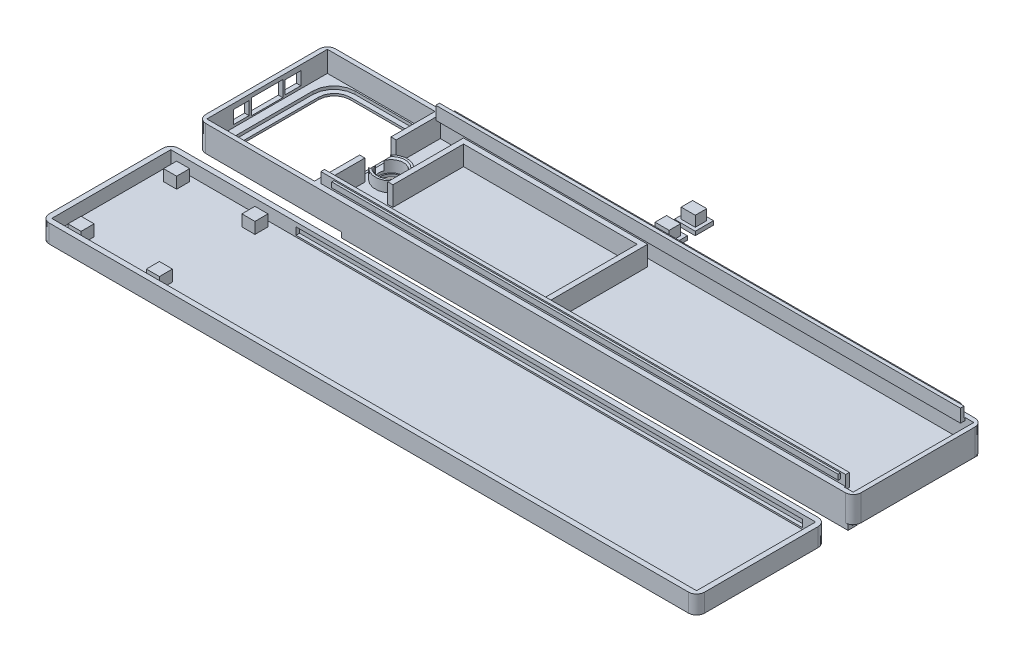
MeetingLight-Enclosure-v11 (Autodesk Fusion 360 design; units mm, degrees)
Autodesk Fusion 360 part; units mm, degrees
sketch "TRAY_Shell" plane through (0, 0, 0) normal (0, 0, 1) x (1, 0, 0)
  line L0 (0, 0) -> (251, 0)
  line L1 (251, 0) -> (251, 49.6)
  line L2 (251, 49.6) -> (0, 49.6)
  line L3 (0, 49.6) -> (0, 0)
  dimension "d26" = 251
  dimension "d27" = 49.6
  constraint coincident L0.start L3.end
  measures "d26" horizontal distance of L0.start L0.end
  measures "d27" vertical distance of L0.start L2.end
extrude "TRAY_Shell (1)" add sketch "TRAY_Shell" along normal blind 7 makes body 1
fillet "TRAY_CornerFillet" radius 3 4 edges at (0, 49.6, 3.5) (251, 49.6, 3.5) (251, 0, 3.5) (0, 0, 3.5) on bodies 1
sketch "TRAY_Cavity" plane through (0, 0, 0) normal (0, 0, 1) x (1, 0, 0)
  line L0 (2, 2) -> (249, 2)
  line L1 (249, 2) -> (249, 47.6)
  line L2 (249, 47.6) -> (2, 47.6)
  line L3 (2, 47.6) -> (2, 2)
  dimension "d32" = 247
  dimension "d33" = 45.6
  dimension "d34" = 2
  dimension "d35" = 2
  constraint horizontal L0
  constraint vertical L1
  measures "d32" horizontal distance of L0.start L0.end
  measures "d33" vertical distance of L0.start L2.end
  measures "d34" horizontal distance of origin L0.start
  measures "d35" vertical distance of origin L0.start
extrude "TRAY_Cavity (1)" cut sketch "TRAY_Cavity" along normal blind 5 from surface at 2 bodies 1
sketch "TRAY_ClampPads" plane through (0, 0, 0) normal (0, 0, 1) x (1, 0, 0)
  line L0 (6.24, 4) -> (11.24, 4)
  line L1 (11.24, 4) -> (11.24, 9)
  line L2 (11.24, 9) -> (6.24, 9)
  line L3 (6.24, 9) -> (6.24, 4)
  line L4 (36.24, 4) -> (41.24, 4)
  line L5 (41.24, 4) -> (41.24, 9)
  line L6 (41.24, 9) -> (36.24, 9)
  line L7 (36.24, 9) -> (36.24, 4)
  line L8 (6.24, 40.6) -> (11.24, 40.6)
  line L9 (11.24, 40.6) -> (11.24, 45.6)
  line L10 (11.24, 45.6) -> (6.24, 45.6)
  line L11 (6.24, 45.6) -> (6.24, 40.6)
  line L12 (36.24, 40.6) -> (41.24, 40.6)
  line L13 (41.24, 40.6) -> (41.24, 45.6)
  line L14 (41.24, 45.6) -> (36.24, 45.6)
  line L15 (36.24, 45.6) -> (36.24, 40.6)
extrude "TRAY_ClampPads (1)" add sketch "TRAY_ClampPads" along normal blind 4.33 from surface at 2 bodies 1
sketch "TRAY_SnapGroove" plane through (0, 0, 0) normal (0, 0, 1) x (1, 0, 0)
  line L0 (50, 0.65) -> (244, 0.65)
  line L1 (244, 0.65) -> (244, 2)
  line L2 (244, 2) -> (50, 2)
  line L3 (50, 2) -> (50, 0.65)
  line L4 (50, 47.6) -> (244, 47.6)
  line L5 (244, 47.6) -> (244, 48.95)
  line L6 (244, 48.95) -> (50, 48.95)
  line L7 (50, 48.95) -> (50, 47.6)
extrude "TRAY_SnapGroove (1)" cut sketch "TRAY_SnapGroove" along normal blind 2.8 from surface at 2.6 bodies 1
sketch "LID_Shell" plane through (0, 0, 0) normal (0, 0, 1) x (1, 0, 0)
  line L0 (0, 0) -> (251, 0)
  line L1 (251, 0) -> (251, 49.6)
  line L2 (251, 49.6) -> (0, 49.6)
  line L3 (0, 49.6) -> (0, 0)
  dimension "d47" = 251
  dimension "d48" = 49.6
  constraint coincident L0.start L3.end
  measures "d47" horizontal distance of L0.start L0.end
  measures "d48" vertical distance of L0.start L2.end
extrude "LID_Shell (1)" add sketch "LID_Shell" along normal blind 10 separate body makes body 2
fillet "LID_CornerFillet" radius 3 4 edges at (0, 49.6, 5) (251, 49.6, 5) (251, 0, 5) (0, 0, 5) on bodies 2
sketch "LID_Cavity" plane through (0, 0, 0) normal (0, 0, 1) x (1, 0, 0)
  line L0 (1.7, 1.7) -> (249.3, 1.7)
  line L1 (249.3, 1.7) -> (249.3, 47.9)
  line L2 (249.3, 47.9) -> (1.7, 47.9)
  line L3 (1.7, 47.9) -> (1.7, 1.7)
  dimension "d53" = 247.6
  dimension "d54" = 46.2
  dimension "d55" = 1.7
  dimension "d56" = 1.7
  measures "d53" horizontal distance of L0.start L0.end
  measures "d54" vertical distance of L0.start L2.end
  measures "d55" horizontal distance of origin L0.start
  measures "d56" vertical distance of origin L0.start
extrude "LID_Cavity (1)" cut sketch "LID_Cavity" along normal blind 8 from surface at 2 bodies 2
sketch "SCREEN_GlassRecess" plane through (0, 0, 0) normal (0, 0, 1) x (1, 0, 0)
  line L0 (6.75, 4.08) -> (40.25, 4.08)
  line L1 (40.25, 4.08) -> (40.25, 45.52)
  line L2 (40.25, 45.52) -> (6.75, 45.52)
  line L3 (6.75, 45.52) -> (6.75, 4.08)
extrude "SCREEN_GlassRecess (1)" cut sketch "SCREEN_GlassRecess" along normal blind 0.84 bodies 2
fillet "SCREEN_GlassRecess_R" radius 6 4 edges at (40.25, 45.52, 0.42) (6.75, 45.52, 0.42) (40.25, 4.08, 0.42) (6.75, 4.08, 0.42) on bodies 2
sketch "SCREEN_BodyOpening" plane through (0, 0, 0) normal (0, 0, 1) x (1, 0, 0)
  line L0 (4.75, 2.25) -> (42.25, 2.25)
  line L1 (42.25, 2.25) -> (42.25, 47.35)
  line L2 (42.25, 47.35) -> (4.75, 47.35)
  line L3 (4.75, 47.35) -> (4.75, 2.25)
extrude "SCREEN_BodyOpening (1)" cut sketch "SCREEN_BodyOpening" along normal blind 1.2 from surface at 0.84 bodies 2
fillet "SCREEN_BodyOpening_R" radius 8 4 edges at (42.25, 2.25, 1.42) (4.75, 2.25, 1.42) (4.75, 47.35, 1.42) (42.25, 47.35, 1.42) on bodies 2
sketch "SCREEN_XStop" plane through (0, 0, 0) normal (0, 0, 1) x (1, 0, 0)
  line L0 (42.94, 1.7) -> (44.94, 1.7)
  line L1 (44.94, 1.7) -> (44.94, 19)
  line L2 (44.94, 19) -> (42.94, 19)
  line L3 (42.94, 19) -> (42.94, 1.7)
  line L4 (42.94, 31) -> (44.94, 31)
  line L5 (44.94, 31) -> (44.94, 47.9)
  line L6 (44.94, 47.9) -> (42.94, 47.9)
  line L7 (42.94, 47.9) -> (42.94, 31)
extrude "SCREEN_XStop (1)" add sketch "SCREEN_XStop" along normal blind 8 from surface at 2 bodies 2
sketch "PAPER_LipFrontWall" plane through (0, 0, 0) normal (0, 0, 1) x (1, 0, 0)
  line L0 (54.99, 0) -> (249.01, 0)
  line L1 (249.01, 0) -> (249.01, 1.5)
  line L2 (249.01, 1.5) -> (54.99, 1.5)
  line L3 (54.99, 1.5) -> (54.99, 0)
extrude "PAPER_LipFrontWall (1)" add sketch "PAPER_LipFrontWall" against normal blind 2 bodies 2
sketch "PAPER_LipFrontShelf" plane through (0, 0, 0) normal (0, 0, 1) x (1, 0, 0)
  line L0 (54.99, 1.5) -> (249.01, 1.5)
  line L1 (249.01, 1.5) -> (249.01, 3.5)
  line L2 (249.01, 3.5) -> (54.99, 3.5)
  line L3 (54.99, 3.5) -> (54.99, 1.5)
extrude "PAPER_LipFrontShelf (1)" add sketch "PAPER_LipFrontShelf" along normal blind 0.8 from surface at -2 bodies 2
sketch "PAPER_LipBackWall" plane through (0, 0, 0) normal (0, 0, 1) x (1, 0, 0)
  line L0 (54.99, 48.1) -> (249.01, 48.1)
  line L1 (249.01, 48.1) -> (249.01, 49.6)
  line L2 (249.01, 49.6) -> (54.99, 49.6)
  line L3 (54.99, 49.6) -> (54.99, 48.1)
extrude "PAPER_LipBackWall (1)" add sketch "PAPER_LipBackWall" against normal blind 2 bodies 2
sketch "PAPER_LipBackShelf" plane through (0, 0, 0) normal (0, 0, 1) x (1, 0, 0)
  line L0 (54.99, 46.1) -> (249.01, 46.1)
  line L1 (249.01, 46.1) -> (249.01, 48.1)
  line L2 (249.01, 48.1) -> (54.99, 48.1)
  line L3 (54.99, 48.1) -> (54.99, 46.1)
extrude "PAPER_LipBackShelf (1)" add sketch "PAPER_LipBackShelf" along normal blind 0.8 from surface at -2 bodies 2
sketch "BAT_PocketWalls" plane through (0, 0, 0) normal (0, 0, 1) x (1, 0, 0)
  line L0 (56.7, 16) -> (58.7, 16)
  line L1 (58.7, 16) -> (58.7, 43.05)
  line L2 (58.7, 43.05) -> (56.7, 43.05)
  line L3 (56.7, 43.05) -> (56.7, 16)
  line L4 (56.7, 43.05) -> (127.2, 43.05)
  line L5 (127.2, 43.05) -> (127.2, 45.05)
  line L6 (127.2, 45.05) -> (56.7, 45.05)
  line L7 (56.7, 45.05) -> (56.7, 43.05)
  line L8 (125.2, 6.55) -> (127.2, 6.55)
  line L9 (127.2, 6.55) -> (127.2, 43.05)
  line L10 (127.2, 43.05) -> (125.2, 43.05)
  line L11 (125.2, 43.05) -> (125.2, 6.55)
  line L12 (56.7, 4.55) -> (127.2, 4.55)
  line L13 (127.2, 4.55) -> (127.2, 6.55)
  line L14 (127.2, 6.55) -> (56.7, 6.55)
  line L15 (56.7, 6.55) -> (56.7, 4.55)
extrude "BAT_PocketWalls (1)" add sketch "BAT_PocketWalls" along normal blind 7.5 from surface at 2 bodies 2
sketch "JOINT_RabbetFoot" plane through (0, 0, 0) normal (0, 0, 1) x (1, 0, 0)
  line L0 (45, 1) -> (246, 1)
  line L1 (246, 1) -> (246, 3.5)
  line L2 (246, 3.5) -> (45, 3.5)
  line L3 (45, 3.5) -> (45, 1)
  line L4 (45, 46.1) -> (246, 46.1)
  line L5 (246, 46.1) -> (246, 48.6)
  line L6 (246, 48.6) -> (45, 48.6)
  line L7 (45, 48.6) -> (45, 46.1)
extrude "JOINT_RabbetFoot (1)" add sketch "JOINT_RabbetFoot" along normal blind 1 from surface at 9 bodies 2
sketch "JOINT_RabbetLip" plane through (0, 0, 0) normal (0, 0, 1) x (1, 0, 0)
  line L0 (45, 2.1) -> (246, 2.1)
  line L1 (246, 2.1) -> (246, 3.5)
  line L2 (246, 3.5) -> (45, 3.5)
  line L3 (45, 3.5) -> (45, 2.1)
  line L4 (45, 46.1) -> (246, 46.1)
  line L5 (246, 46.1) -> (246, 47.5)
  line L6 (246, 47.5) -> (45, 47.5)
  line L7 (45, 47.5) -> (45, 46.1)
extrude "JOINT_RabbetLip (1)" add sketch "JOINT_RabbetLip" along normal blind 4 from surface at 10 bodies 2
sketch "IO_USB" plane through (0, 0, 0) normal (0, 0, 1) x (1, 0, 0)
  line L0 (-0.5, 18.8) -> (2, 18.8)
  line L1 (2, 18.8) -> (2, 30.8)
  line L2 (2, 30.8) -> (-0.5, 30.8)
  line L3 (-0.5, 30.8) -> (-0.5, 18.8)
  dimension "d97" = 12
  measures "d97" vertical distance of L0.start L2.end
extrude "IO_USB (1)" cut sketch "IO_USB" along normal blind 6 from surface at 2.5 bodies 2
sketch "IO_Btn1" plane through (0, 0, 0) normal (0, 0, 1) x (1, 0, 0)
  line L0 (-0.5, 11.9) -> (2, 11.9)
  line L1 (2, 11.9) -> (2, 17.9)
  line L2 (2, 17.9) -> (-0.5, 17.9)
  line L3 (-0.5, 17.9) -> (-0.5, 11.9)
  dimension "d101" = 6
  measures "d101" vertical distance of L0.start L2.end
extrude "IO_Btn1 (1)" cut sketch "IO_Btn1" along normal blind 5 from surface at 3 bodies 2
sketch "IO_Btn2" plane through (0, 0, 0) normal (0, 0, 1) x (1, 0, 0)
  line L0 (-0.5, 31.7) -> (2, 31.7)
  line L1 (2, 31.7) -> (2, 37.7)
  line L2 (2, 37.7) -> (-0.5, 37.7)
  line L3 (-0.5, 37.7) -> (-0.5, 31.7)
  dimension "d105" = 6
  measures "d105" vertical distance of L0.start L2.end
extrude "IO_Btn2 (1)" cut sketch "IO_Btn2" along normal blind 5 from surface at 3 bodies 2
sketch "CAP1_Base" plane through (0, 0, 0) normal (0, 0, 1) x (1, 0, 0)
  line L0 (116, 116.5) -> (124, 116.5)
  line L1 (124, 116.5) -> (124, 123.5)
  line L2 (124, 123.5) -> (116, 123.5)
  line L3 (116, 123.5) -> (116, 116.5)
extrude "CAP1_Base (1)" add sketch "CAP1_Base" along normal blind 1.5 separate body makes body 3
sketch "CAP1_Stem" plane through (0, 0, 0) normal (0, 0, 1) x (1, 0, 0)
  line L0 (117.3, 117.8) -> (122.7, 117.8)
  line L1 (122.7, 117.8) -> (122.7, 122.2)
  line L2 (122.7, 122.2) -> (117.3, 122.2)
  line L3 (117.3, 122.2) -> (117.3, 117.8)
extrude "CAP1_Stem (1)" add sketch "CAP1_Stem" along normal blind 4 from surface at 1.5 bodies 3
sketch "CAP2_Base" plane through (0, 0, 0) normal (0, 0, 1) x (1, 0, 0)
  line L0 (116, 126.5) -> (124, 126.5)
  line L1 (124, 126.5) -> (124, 133.5)
  line L2 (124, 133.5) -> (116, 133.5)
  line L3 (116, 133.5) -> (116, 126.5)
extrude "CAP2_Base (1)" add sketch "CAP2_Base" along normal blind 1.5 separate body makes body 4
sketch "CAP2_Stem" plane through (0, 0, 0) normal (0, 0, 1) x (1, 0, 0)
  line L0 (117.3, 127.8) -> (122.7, 127.8)
  line L1 (122.7, 127.8) -> (122.7, 132.2)
  line L2 (122.7, 132.2) -> (117.3, 132.2)
  line L3 (117.3, 132.2) -> (117.3, 127.8)
extrude "CAP2_Stem (1)" add sketch "CAP2_Stem" along normal blind 4 from surface at 1.5 bodies 4
move_body "LAYOUT_MoveLid" bodies 2 to x (1, 0, 0) y (0, 1, 0) z (0, 0, 1) at (0, 60, 0)
sketch "JOINT_SnapRib" plane through (0, 0, 0) normal (0, 0, 1) x (1, 0, 0)
  line L0 (50, 61.25) -> (244, 61.25)
  line L1 (244, 61.25) -> (244, 62.3)
  line L2 (244, 62.3) -> (50, 62.3)
  line L3 (50, 62.3) -> (50, 61.25)
  line L4 (50, 107.3) -> (244, 107.3)
  line L5 (244, 107.3) -> (244, 108.35)
  line L6 (244, 108.35) -> (50, 108.35)
  line L7 (50, 108.35) -> (50, 107.3)
extrude "JOINT_SnapRib (1)" add sketch "JOINT_SnapRib" along normal blind 2 from surface at 11.5 bodies 2
sketch "PIR_CanHole" plane through (0, 0, 0) normal (0, 0, 1) x (1, 0, 0)
  circle A0 centre (49.25, 84.8) radius 4.245
  dimension "d127" = 8.49
  measures "d127" diameter of A0
extrude "PIR_CanHole (1)" cut sketch "PIR_CanHole" along normal blind 2 bodies 2
sketch "PIR_BrimCounterbore" plane through (0, 0, 0) normal (0, 0, 1) x (1, 0, 0)
  circle A0 centre (49.25, 84.8) radius 4.75
  dimension "d130" = 9.5
  measures "d130" diameter of A0
extrude "PIR_BrimCounterbore (1)" cut sketch "PIR_BrimCounterbore" along normal blind 1 from surface at 1 bodies 2
sketch "PIR_CollarBoss" plane through (0, 0, 0) normal (0, 0, 1) x (1, 0, 0)
  circle A0 centre (49.25, 84.8) radius 6.15
  dimension "d139" = 12.3
  measures "d139" diameter of A0
extrude "PIR_CollarBoss (1)" add sketch "PIR_CollarBoss" along normal blind 4 from surface at 2 bodies 2
sketch "PIR_CollarBore" plane through (0, 0, 0) normal (0, 0, 1) x (1, 0, 0)
  circle A0 centre (49.25, 84.8) radius 4.75
  dimension "d143" = 9.5
  measures "d143" diameter of A0
extrude "PIR_CollarBore (1)" cut sketch "PIR_CollarBore" along normal blind 4 from surface at 2 bodies 2
sketch "PIR_CollarSlotXp" plane through (0, 0, 0) normal (0, 0, 1) x (1, 0, 0)
  line L0 (53.7, 80.56) -> (55.7, 80.56)
  line L1 (55.7, 80.56) -> (55.7, 89.04)
  line L2 (55.7, 89.04) -> (53.7, 89.04)
  line L3 (53.7, 89.04) -> (53.7, 80.56)
extrude "PIR_CollarSlotXp (1)" cut sketch "PIR_CollarSlotXp" along normal blind 4 from surface at 2 bodies 2
sketch "PIR_CollarSlotXn" plane through (0, 0, 0) normal (0, 0, 1) x (1, 0, 0)
  line L0 (42.8, 80.56) -> (44.8, 80.56)
  line L1 (44.8, 80.56) -> (44.8, 89.04)
  line L2 (44.8, 89.04) -> (42.8, 89.04)
  line L3 (42.8, 89.04) -> (42.8, 80.56)
extrude "PIR_CollarSlotXn (1)" cut sketch "PIR_CollarSlotXn" along normal blind 4 from surface at 2 bodies 2
chamfer "PIR_CollarLeadIn" distance 0.6 angle 45 6 edges at (44.8, 81.8493, 6) (44.8, 87.7507, 6) (49.25, 80.05, 6) (49.25, 89.55, 6) (53.7, 81.8493, 6) (53.7, 87.7507, 6) on bodies 2
equation "enc_len = 251 mm" comment "Shell: overall length"
equation "enc_wid = 49.6 mm" comment "Shell: overall width"
equation "wall = 2.0 mm" comment "Shell: nominal wall thickness"
equation "tol = 0.3 mm" comment "Shell: fit clearance/tolerance"
equation "corner_r = 3.0 mm" comment "Shell: outer corner radius"
equation "tray_depth = 7 mm" comment "Shell: back tray total depth"
equation "lid_depth = 10.0 mm" comment "Shell: front lid body depth"
equation "scr_pocket_w = 38.0 mm" comment "Screen: pocket width (X)"
equation "scr_pocket_h = 45.6 mm" comment "Screen: pocket height (Y)"
equation "scr_pocket_depth = 8.0 mm" comment "Screen: pocket depth"
equation "glass_recess_r = 6 mm" comment "Screen: glass recess corner radius"
equation "scr_center_x = 23.5 mm" comment "Screen: pocket center X"
equation "scr_center_y = 24.8 mm" comment "Screen: pocket center Y"
equation "bat_pocket_len = 66.5 mm" comment "Battery: inner pocket length (X)"
equation "bat_pocket_wid = 36.5 mm" comment "Battery: inner pocket width (Y)"
equation "bat_center_x = 90.95 mm" comment "Battery: pocket center X"
equation "bat_center_y = 24.8 mm" comment "Battery: pocket center Y"
equation "pir_center_x = 49.25 mm" comment "PIR: aperture center X"
equation "pir_center_y = 24.8 mm" comment "PIR: aperture center Y"
equation "snap_catch = 0.7 mm" comment "Joint: snap rib/groove catch depth"
equation "rabbet_lip_depth = 4.0 mm" comment "Joint: rabbet lip depth"
equation "clamp_pad_h = 4.33 mm" comment "Joint: screen clamp pad height"
equation "io_usb_h = 12.0 mm" comment "IO: USB-C cutout height (Y)"
equation "io_btn_h = 6.0 mm" comment "IO: button cutout height (Y)"
equation "d26 = enc_len"
equation "d27 = enc_wid"
equation "d28 = tray_depth"
equation "d31 = corner_r"
equation "d32 = enc_len - 2 * wall"
equation "d33 = enc_wid - 2 * wall"
equation "d34 = wall"
equation "d35 = wall"
equation "d36 = wall"
equation "d37 = tray_depth - wall"
equation "d41 = wall"
equation "d42 = clamp_pad_h"
equation "d47 = enc_len"
equation "d48 = enc_wid"
equation "d49 = lid_depth"
equation "d52 = corner_r"
equation "d53 = enc_len - 3.4 mm"
equation "d54 = enc_wid - 3.4 mm"
equation "d58 = lid_depth - 2 mm"
equation "d63 = glass_recess_r"
equation "d68 = screen_opening_r"
equation "d70 = lid_depth - 2 mm"
equation "d92 = rabbet_lip_depth"
equation "d97 = io_usb_h"
equation "d101 = io_btn_h"
equation "d105 = io_btn_h"
equation "d109 = cap_base_h"
equation "d111 = cap_base_h"
equation "d114 = cap_base_h"
equation "d116 = cap_base_h"
equation "screen_opening_r = 8 mm" comment "Screen: body-opening (larger pocket) corner radius"
equation "cap_base_h = 1.5 mm" comment "Caps: top-hat base flange height (was 2.5; reduce to clear screen buttons)"
equation "pir_can_dia = 8.19 mm" comment "PIR: metal can diameter (press-through)"
equation "pir_brim_dia = 9.2 mm" comment "PIR: can base brim/flange diameter (counterbore stop)"
equation "pir_brim_depth = 1.0 mm" comment "PIR: brim counterbore depth from cavity face (~brim height)"
equation "d127 = pir_can_dia + tol"
equation "d128 = wall"
equation "d130 = pir_brim_dia + tol"
equation "d131 = wall - pir_brim_depth"
equation "d132 = pir_brim_depth"
equation "pir_pcb_w = 10.0 mm" comment "PIR: sensor PCB width (slotted axis, along X)"
equation "pir_pcb_h = 7.88 mm" comment "PIR: sensor PCB height, can->pin (along Y)"
equation "pir_pcb_t = 1.0 mm" comment "PIR: sensor PCB thickness"
equation "pir_collar_wall = 1.4 mm" comment "PIR: guide collar/tube wall thickness"
equation "pir_collar_h = 4.0 mm" comment "PIR: guide collar height above cavity floor (< battery ribs)"
equation "d139 = pir_brim_dia + tol + 2 * pir_collar_wall"
equation "d140 = wall"
equation "d141 = pir_collar_h"
equation "d143 = pir_brim_dia + tol"
equation "d144 = wall"
equation "d145 = pir_collar_h"
equation "d147 = wall"
equation "d148 = pir_collar_h"
equation "d150 = wall"
equation "d151 = pir_collar_h"
equation "pir_chamfer = 0.6 mm" comment "PIR: collar/slot top lead-in chamfer"
equation "d154 = pir_chamfer"
named bodies: "Back Tray", "Front Lid", "ButtonCap_1", "ButtonCap_2"
